Autodesk Inventor part; units mm, degrees
(part 2 of 2)
  arc A620 (20.4911, 0.6052) -> (20.4754, 1.0044) centre (0, 0) ccw
  arc A621 (20.3804, 2.2111) -> (20.3335, 2.6078) centre (0, 0) ccw
  arc A622 (20.1441, 3.8033) -> (20.0662, 4.1951) centre (0, 0) ccw
  arc A623 (19.7836, 5.372) -> (19.6752, 5.7565) centre (0, 0) ccw
  arc A624 (19.3011, 6.9077) -> (19.1629, 7.2825) centre (0, 0) ccw
  arc A625 (18.6997, 8.4007) -> (18.5324, 8.7635) centre (0, 0) ccw
  arc A626 (17.9829, 9.842) -> (17.7877, 10.1905) centre (0, 0) ccw
  arc A627 (17.1553, 11.2226) -> (16.9334, 11.5547) centre (0, 0) ccw
  arc A628 (16.2219, 12.534) -> (15.9746, 12.8477) centre (0, 0) ccw
  arc A629 (15.1885, 13.7681) -> (14.9173, 14.0614) centre (0, 0) ccw
  arc A630 (14.0614, 14.9173) -> (13.7681, 15.1885) centre (0, 0) ccw
  arc A631 (12.8477, 15.9746) -> (12.534, 16.2219) centre (0, 0) ccw
  arc A632 (11.5547, 16.9334) -> (11.2226, 17.1553) centre (0, 0) ccw
  arc A633 (10.1905, 17.7877) -> (9.842, 17.9829) centre (0, 0) ccw
  arc A634 (8.7635, 18.5324) -> (8.4007, 18.6997) centre (0, 0) ccw
  arc A635 (7.2825, 19.1629) -> (6.9077, 19.3011) centre (0, 0) ccw
  arc A636 (5.7565, 19.6752) -> (5.372, 19.7836) centre (0, 0) ccw
  arc A637 (4.1951, 20.0662) -> (3.8033, 20.1441) centre (0, 0) ccw
  arc A638 (2.6078, 20.3335) -> (2.2111, 20.3804) centre (0, 0) ccw
  arc A639 (1.0044, 20.4754) -> (0.6052, 20.4911) centre (0, 0) ccw
  line L0 (-22.5, 0) -> (22.5, 0)
  line L1 (0, -22.5) -> (0, 22.5)
  point P0 (0, 0)
  constraints: 960 point on circle, 480 centre point, 4 end point, 2 horizontal alignment, 2 vertical alignment, 476 other
extrude "Extrusion1" add sketch "Sketch1" against normal blind 3
sketch "Sketch2" plane through (0, 0, 0) normal (0, 0, 1) x (1, 0, 0)
  circle A0 centre (0, 14) radius 1.25
  circle A1 centre (-12.1244, -7) radius 1.25
  circle A2 centre (12.1244, -7) radius 1.25
  point P0 (0, 0)
  dimension "d3" = 2.5
  dimension "d6" = 360
  dimension "d8" = 14
  constraints: 3 centre point, 1 horizontal alignment, 7 other
  measures "d3" diameter of A0
  measures "d8" distance of point (0, 0) A0.centre
extrude "Extrusion2" cut sketch "Sketch2" against normal through all
sketch "Sketch3" plane through (0, 0, 0) normal (0, 0, 1) x (1, 0, 0)
  circle A0 centre (0, 0) radius 18.25
  dimension "d11" = 36.5
  constraints: 1 centre point, 1 coincident
  measures "d11" diameter of A0
extrude "Extrusion3" cut sketch "Sketch3" against normal blind 0.75
sketch "Sketch4" plane through (0, 0, -3) normal (0, 0, -1) x (-1, 0, 0)
  circle A0 centre (0, 0) radius 18.25 projected
extrude "Extrusion4" cut sketch "Sketch4" against normal blind 0.75
sketch "Sketch5" plane through (0, 0, -2.25) normal (0, 0, -1) x (-1, 0, 0)
  circle A0 centre (0, 14) radius 1.25 projected
  circle A1 centre (-12.1244, -7) radius 1.25 projected
  circle A2 centre (12.1244, -7) radius 1.25 projected
  arc A3 (-4.1783, 13.2229) -> (4.1783, 13.2229) centre (0, 14) ccw
  arc A4 (-9.3622, -10.23) -> (-13.5405, -2.9929) centre (-12.1244, -7) ccw
  arc A5 (13.5405, -2.9929) -> (9.3622, -10.23) centre (12.1244, -7) ccw
  arc A6 (-4.1783, 13.2229) -> (-7.007, 14.6617) centre (-6.1446, 12.8571) ccw
  arc A7 (-7.007, 14.6617) -> (-16.2009, -1.2626) centre (0, 0) ccw
  arc A8 (-16.2009, -1.2626) -> (-13.5405, -2.9929) centre (-14.2069, -1.1072) ccw
  circle A9 centre (0, 0) radius 18.25 projected
  arc A10 (9.1939, -13.3991) -> (9.3622, -10.23) centre (8.0623, -11.75) ccw
  arc A11 (-9.1939, -13.3991) -> (9.1939, -13.3991) centre (0, 0) ccw
  arc A12 (-9.3622, -10.23) -> (-9.1939, -13.3991) centre (-8.0623, -11.75) ccw
  arc A13 (7.007, 14.6617) -> (4.1783, 13.2229) centre (6.1446, 12.8571) ccw
  arc A14 (16.2009, -1.2626) -> (7.007, 14.6617) centre (0, 0) ccw
  arc A15 (13.5405, -2.9929) -> (16.2009, -1.2626) centre (14.2069, -1.1072) ccw
  point P0 (9.3622, -10.23)
  point P1 (13.5405, -2.9929)
  point P2 (4.1783, 13.2229)
  dimension "d16" = 3
  dimension "d19" = 360
  dimension "d21" = 2
  dimension "d22" = 2
  dimension "d25" = 360
  constraints: 24 point on circle, 12 centre point, 4 tangent, 2 concentric, 1 equal radius, 44 other
  measures "d16" radial gap between concentric circles of A0 A3
  measures "d21" radial gap between concentric circles of A9 A7
  measures "d22" radius of A6
extrude "Extrusion5" cut sketch "Sketch5" against normal through all contours A3 A13 A14 A15 A5 A10 A11 A12 A4 A8 A7 A6
body "Solid1"
